naze32 support (Autodesk Fusion 360 design; units mm, degrees)
Autodesk Fusion 360 part; units mm, degrees
sketch "base" plane through (0, 0, 0) normal (0, 0, 1) x (1, 0, 0)
  line L0 (14.5, 46.5) -> (-14.5, 46.5)
  line L1 (-14.5, 46.5) -> (-14.5, -46.5)
  line L2 (-14.5, -46.5) -> (14.5, -46.5)
  line L3 (14.5, -46.5) -> (14.5, 46.5)
  line L4 (14.5, 46.5) -> (-14.5, -46.5) construction
  line L5 (-14.5, 46.5) -> (14.5, -46.5) construction
  line L6 (22.5, 12.5) -> (-22.5, -12.5) construction
  line L7 (-22.5, 12.5) -> (22.5, -12.5) construction
  line L8 (0, 0) -> (0, 38.1)
  line L9 (0, 0) -> (0, -38.1)
  circle A0 centre (0, 38.1) radius 2
  circle A1 centre (0, -38.1) radius 2
  line L10 (21, -21) -> (-21, -21)
  line L11 (-21, -21) -> (-21, 21)
  line L12 (-21, 21) -> (21, 21)
  line L13 (21, 21) -> (21, -21)
  line L14 (21, -21) -> (-21, 21) construction
  line L15 (-21, -21) -> (21, 21) construction
  line L16 (23.2, -23.2) -> (-23.2, -23.2)
  line L17 (-23.2, -23.2) -> (-23.2, 23.2)
  line L18 (-23.2, 23.2) -> (23.2, 23.2)
  line L19 (23.2, 23.2) -> (23.2, -23.2)
  line L20 (14.5, 34.0288) -> (12.0174, 34.0288)
  line L21 (12.0174, 34.0288) -> (12.0174, 23.2)
  line L22 (12.0174, 23.2) -> (14.5, 23.2)
  line L23 (14.5, 23.2) -> (14.5, 34.0288)
  line L24 (-12.0174, 34.0288) -> (-12.0174, 23.2)
  line L25 (-14.5, 34.0288) -> (-12.0174, 34.0288)
  line L26 (-12.0174, 23.2) -> (-14.5, 23.2)
  line L27 (-14.5, 23.2) -> (-14.5, 34.0288)
  line L28 (23.2, 0) -> (-23.2, 0)
  line L29 (12.0174, -34.0288) -> (12.0174, -23.2)
  line L30 (14.5, -34.0288) -> (12.0174, -34.0288)
  line L31 (12.0174, -23.2) -> (14.5, -23.2)
  line L32 (14.5, -23.2) -> (14.5, -34.0288)
  line L33 (-12.0174, -34.0288) -> (-12.0174, -23.2)
  line L34 (-14.5, -34.0288) -> (-12.0174, -34.0288)
  line L35 (-14.5, -23.2) -> (-14.5, -34.0288)
  line L36 (-12.0174, -23.2) -> (-14.5, -23.2)
  dimension "d1" = 29
  dimension "d2" = 93
  dimension "d3" = 45
  dimension "d4" = 25
  dimension "d7" = 4
  dimension "d8" = 4
  dimension "d35" = 38.1
  dimension "d36" = 38.1
  dimension "d37" = 42
  dimension "d38" = 42
  dimension "d39" = -2.2
  dimension "d55" = 2.4826
  constraint horizontal L0
  constraint perpendicular L0 L1
  constraint parallel L0 L2
  constraint parallel L1 L3
  constraint coincident L4 L8.start
  constraint coincident L5 L8.start
  constraint coincident L8.start L9.start
  constraint coincident L6 L8.start
  constraint coincident L7 L8.start
  constraint coincident L8.end A0.centre
  constraint coincident L9.end A1.centre
  constraint horizontal L10
  constraint perpendicular L10 L11
  constraint parallel L10 L12
  constraint parallel L11 L13
  constraint coincident L14 L8.start
  constraint coincident L15 L8.start
  constraint horizontal L20
  constraint vertical L21
  constraint horizontal L22
  constraint vertical L23
  constraint coincident L3 L20.start
  constraint symmetric L8 L20.start L25.start
  constraint symmetric L8 L20.end L24.start
  constraint symmetric L8 L21.end L24.end
  constraint symmetric L8 L22.end L26.end
  constraint midpoint L19 L28.start
  constraint midpoint L17 L28.end
  constraint symmetric L20.start L28 L30.start
  constraint symmetric L20.end L28 L29.start
  constraint symmetric L21.end L28 L29.end
  constraint symmetric L22.end L28 L31.end
  constraint symmetric L24.start L28 L33.start
  constraint symmetric L24.end L28 L33.end
  constraint symmetric L25.start L28 L34.start
  constraint symmetric L26.end L28 L35.start
  measures "d1" distance of L1.end L2.end
  measures "d2" distance of L0.end L1.end
  measures "d3" distance of L6.end L7.end
  measures "d4" distance of L7.start L6.end
  measures "d7" diameter of A0
  measures "d8" diameter of A1
  measures "d35" distance of L8.start L8.end
  measures "d36" distance of L8.start L9.end
  measures "d37" distance of L11.end L12.end
  measures "d38" distance of L10.end L11.end
  measures "d55" distance of L20.start L20.end
extrude "Extrude1" add sketch "base" along normal blind 2.4 contours L0 L1 L3 L18 L20 L21 L24 L25 | L3 L18 L20 L21 L22 L23 | L1 L18 L24 L25 L26 L27 | L3 L8 L12 L18 L22 | L1 L8 L12 L18 L26 | L3 L8 L12 L28 | L1 L8 L12 L28 | L3 L9 L10 L28 | L1 L9 L10 L28 | L3 L9 L10 L16 L31 | L1 L9 L10 L16 L36 | L3 L16 L29 L30 L31 L32 | L1 L16 L33 L34 L35 L36 | L1 L2 L3 L16 L29 L30 L33 L34
ref_plane "WorkPlane1" through (0, 0, 2.4) normal (0, 0, 1) x (1, 0, 0)
sketch "Sketch4" plane through (0, 0, 0) normal (1, 0, 0) x (0, 1, 0)
  line L0 (0, 0) -> (0, 18.158)
  spline S0 degree 5 poles (30.0169, 12.3954) (30.115, 12.1372) (30.2812, 11.6469) (30.4403, 10.9895) (30.4713, 10.2698) (30.2114, 9.6276) (29.6709, 9.2232) (28.8914, 9.0138) (27.9508, 8.919) (26.9536, 8.8356) (26.0129, 8.6625) (25.2351, 8.3225) (24.7041, 7.7842) (24.4635, 7.0881) (24.526, 6.3227) (24.8851, 5.5971) (25.5246, 5.0142) (26.4293, 4.6453) (27.5853, 4.5365) (28.9805, 4.7143) (30.6053, 5.1912) (32.0832, 5.8146) (33.29, 6.4175) (34.138, 6.8793) (34.5729, 7.1252) knots 0 0 0 0 0 0 0.05 0.1 0.15 0.2 0.25 0.3 0.35 0.4 0.45 0.5 0.55 0.6 0.65 0.7 0.75 0.8 0.85 0.9 0.95 1 1 1 1 1 1
  line L1 (30.0169, 12.3954) -> (34.9177, 12.3954)
  line L2 (34.9177, 12.3954) -> (34.5729, 7.1252)
  line L3 (29.0791, 14.8624) -> (30.9546, 9.9284)
  line L4 (32.2002, 5.7836) -> (36.9455, 8.4668)
  line L5 (14.3, 2.4) -> (-14.3, 2.4)
  line L6 (-25.5, 2.4) -> (-14.3, 2.4)
  line L7 (25.5, 2.4) -> (14.3, 2.4)
  line L8 (-30.0169, 12.3954) -> (-34.9177, 12.3954)
  line L9 (-34.9177, 12.3954) -> (-34.5729, 7.1252)
  spline S1 degree 5 poles (-30.0169, 12.3954) (-30.115, 12.1372) (-30.2812, 11.6469) (-30.4403, 10.9895) (-30.4713, 10.2698) (-30.2114, 9.6276) (-29.6709, 9.2232) (-28.8914, 9.0138) (-27.9508, 8.919) (-26.9536, 8.8356) (-26.0129, 8.6625) (-25.2351, 8.3225) (-24.7041, 7.7842) (-24.4635, 7.0881) (-24.526, 6.3227) (-24.8851, 5.5971) (-25.5246, 5.0142) (-26.4293, 4.6453) (-27.5853, 4.5365) (-28.9805, 4.7143) (-30.6053, 5.1912) (-32.0832, 5.8146) (-33.29, 6.4175) (-34.138, 6.8793) (-34.5729, 7.1252) knots 0 0 0 0 0 0 0.05 0.1 0.15 0.2 0.25 0.3 0.35 0.4 0.45 0.5 0.55 0.6 0.65 0.7 0.75 0.8 0.85 0.9 0.95 1 1 1 1 1 1
  line L10 (-29.0791, 14.8624) -> (-30.9546, 9.9284)
  line L11 (-32.2002, 5.7836) -> (-36.9455, 8.4668)
  point P0 (29.4258, 9.1939)
  point P1 (25.2392, 8.2334)
  point P2 (24.9437, 5.6476)
  point P3 (-29.4258, 9.1939)
  point P4 (-25.2392, 8.2334)
  point P5 (-24.9437, 5.6476)
  constraint coincident L0.start origin
  constraint vertical L0
  constraint horizontal L1
  constraint midpoint S0.start L3
  constraint midpoint S0.end L4
  constraint symmetric L0 S0.start L8.start
  constraint symmetric L0 P0 P3
  constraint symmetric L0 P1 P4
  constraint symmetric L0 P2 P5
  constraint symmetric L0 S0.end L9.end
  constraint symmetric L0 L1.end L8.end
  constraint symmetric L0 L3.start L10.start
  constraint symmetric L0 L3.end L10.end
  constraint symmetric L0 L4.start L11.start
  constraint symmetric L0 L4.end L11.end
extrude "Extrude8" add sketch "base" along normal blind 12 contours L3 L12 L13 L18 L19 L28 | L3 L8 L12 L18 L22 | L1 L8 L12 L18 L26 | L1 L11 L12 L17 L18 L28 | L3 L10 L13 L16 L19 L28 | L1 L10 L11 L16 L17 L28 | L3 L9 L10 L16 L31 | L1 L9 L10 L16 L36
extrude "Extrude9" add sketch "base" along normal blind 2.4 contours L1 L11 L12 L28 | L1 L10 L11 L28
extrude "Extrude10" add sketch "base" along normal blind 2.4 contours L3 L12 L13 L28 | L3 L10 L13 L28
sketch "Sketch5" plane through (0, 0, 0) normal (1, 0, 0) x (0, 1, 0)
  line L0 (4, 11.4) -> (16, 11.4)
  line L1 (16, 11.4) -> (16, 5.4)
  line L2 (16, 5.4) -> (4, 5.4)
  line L3 (4, 5.4) -> (4, 11.4)
  line L4 (20, 11.9472) -> (20, 0)
  line L5 (0, 0) -> (20, 0)
  line L6 (0, 0) -> (0, 14.0292)
  dimension "d46" = 12
  dimension "d47" = 6
  dimension "d48" = 12
  dimension "d49" = 12
  dimension "d50" = 5.4
  dimension "d54" = 4
  constraint vertical L4
  constraint coincident L5.start L6.start
  constraint perpendicular L4 L5
  constraint perpendicular L5 L6
  measures "d46" distance of L1 L3
  measures "d47" distance of L0 L2
  measures "d48" distance of L1.end L2.end
  measures "d49" distance of L1.end L2.end
  measures "d50" distance of L2 L5
  measures "d54" distance of L3 L6
extrude "Extrude11" cut sketch "Sketch5" along normal blind 28
extrude "Extrude12" add sketch "base" along normal blind 12 contours L3 L18 L20 L21 L22 L23 | L1 L18 L24 L25 L26 L27 | L3 L16 L29 L30 L31 L32 | L1 L16 L33 L34 L35 L36
extrude "Extrude13" cut sketch "Sketch4" along normal through all and the other way through all
chamfer "Chamfer2" distance 2.2 angle 45 8 edges at (12.0174, -23.2, 7.2) (14.5, -23.2, 6) (-12.0174, -23.2, 7.2) (-14.5, -23.2, 6) (-14.5, 23.2, 6) (-12.0174, 23.2, 7.2) (12.0174, 23.2, 7.2) (14.5, 23.2, 6)
fillet "Fillet4" radius 8 4 edges at (14.5, -46.5, 1.2) (-14.5, -46.5, 1.2) (14.5, 46.5, 1.2) (-14.5, 46.5, 1.2)
fillet "Fillet5" radius 1 4 edges at (-13.2587, 34.0288, 6.8232) (13.2587, 34.0288, 6.8232) (13.2587, -34.0288, 6.8232) (-13.2587, -34.0288, 6.8232)
